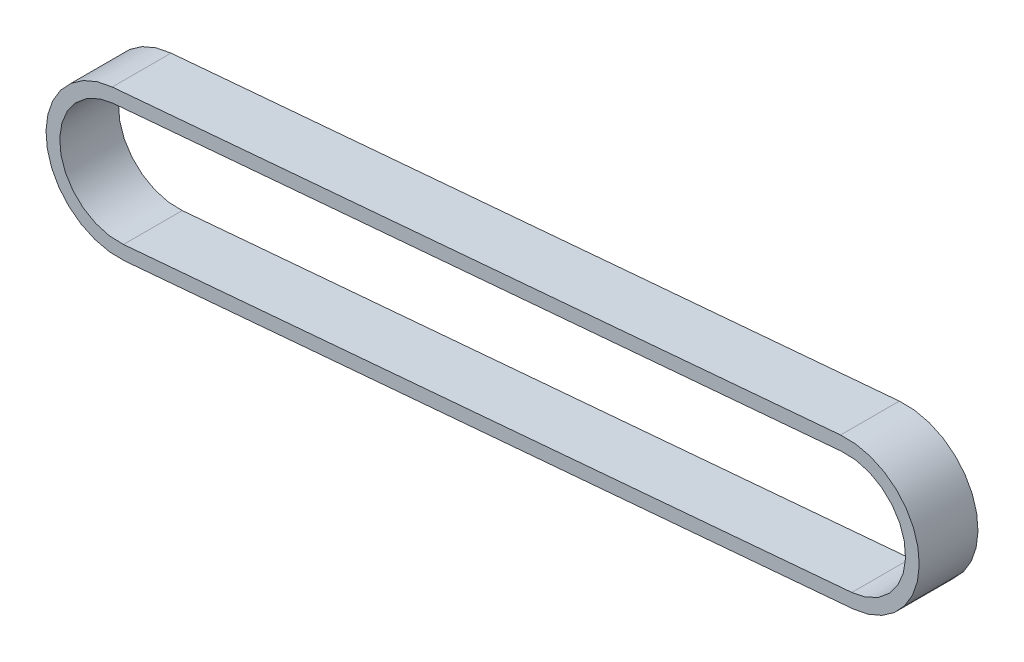
# Autodesk Inventor part: ремень оси y моторный
Saved by Autodesk Inventor 2017 (Build 210142000, 142)
## iProperties
Part Number: ремень оси y моторный
Material: Типовые
Document SubType Name: Modeling
Designer: Max
Mass: 1.60778 g
Surface Area: 28.3276 cm^2
Volume: 1.60778 cm^3
Density: 1 g/cm^3
Appearance: Резина — черная — версия 1.1
Author: Max
Autodesk Inventor part; units mm, degrees
ref_plane "YZ Plane" through (0, 0, 0) normal (1, 0, 0) x (0, 1, 0)
ref_plane "XZ Plane" through (0, 0, 0) normal (0, 1, 0) x (-1, 0, 0)
ref_plane "XY Plane" through (0, 0, 0) normal (0, 0, 1) x (1, 0, 0)
sketch "Эскиз1" plane through (0, 0, 0) normal (0, 0, 1) x (1, 0, 0)
  arc A0 (0.5156, -5.9778) -> (-0.5156, 5.9778) centre (0, 0) ccw
  arc A1 (0.6359, -7.3726) -> (-0.6359, 7.3726) centre (0, 0) ccw
  circle A2 centre (-74.3766, -6.4146) radius 2 projected
  arc A3 (-74.8921, -0.4368) -> (-73.861, -12.3924) centre (-74.3766, -6.4146) ccw
  arc A4 (-75.0124, 0.9581) -> (-73.7407, -13.7872) centre (-74.3766, -6.4146) ccw
  line L0 (-75.0124, 0.9581) -> (-0.6359, 7.3726)
  line L1 (0.6359, -7.3726) -> (-73.7407, -13.7872)
  line L2 (-73.861, -12.3924) -> (0.5156, -5.9778)
  line L3 (-0.5156, 5.9778) -> (-74.8921, -0.4368)
  dimension "d0" = 12
  dimension "d1" = 1.4
  dimension "d2" = 12
  dimension "d3" = 1.4
  constraints: 8 end point, 8 point on circle, 8 tangent, 4 centre point, 4 coincident
  measures "d0" diameter of A0
  measures "d1" radial gap between concentric circles of A0 A1
  measures "d2" diameter of A3
  measures "d3" radial gap between concentric circles of A4 A3
extrude "Выдавливание1" add sketch "Эскиз1" against normal blind 6 contours L1 A4 L0 A1
